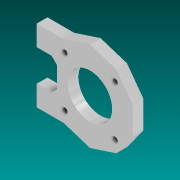
# Autodesk Inventor part: motorFrame
Saved by Autodesk Inventor 2020.2 (Build 242310000, 310)
## iProperties
Created: 2020-05-19
Part Number: motorFrame
Material: Aluminum 6061
Document SubType Name: Modeling
Designer: Svend
Density: 2.7 g/cm^3
Appearance: Aluminum - Polished
Author: Svend
Autodesk Inventor part; units mm, degrees
ref_plane "YZ Plane" through (0, 0, 0) normal (1, 0, 0) x (0, 1, 0)
ref_plane "XZ Plane" through (0, 0, 0) normal (0, 1, 0) x (-1, 0, 0)
ref_plane "XY Plane" through (0, 0, 0) normal (0, 0, 1) x (1, 0, 0)
ref_plane "Work Plane1" through (0, 0, 0) normal (0, 0, 1) x (1, 0, 0)
sketch "Sketch1" plane through (0, 0, 0) normal (0, 0, 1) x (1, 0, 0)
  circle A0 centre (0, 0) radius 21 projected
  circle A1 centre (23.57, -23.57) radius 2 projected
  circle A2 centre (23.57, 23.57) radius 2 projected
  circle A3 centre (-23.57, -23.57) radius 2.5 projected
  circle A4 centre (-23.57, 23.57) radius 2 projected
  circle A5 centre (-23.57, -23.57) radius 2 projected
  circle A6 centre (0, 0) radius 19 projected
  circle A7 centre (-23.57, 23.57) radius 2.5 projected
  circle A8 centre (-23.57, -23.57) radius 2.5 projected
  arc A9 (-29.95, -24.95) -> (-24.95, -29.95) centre (-24.95, -24.95) ccw projected
  line L0 (24.95, -29.95) -> (-24.95, -29.95) projected
  arc A10 (24.95, -29.95) -> (29.95, -24.95) centre (24.95, -24.95) ccw projected
  line L1 (29.95, 24.95) -> (29.95, -24.95) projected
  arc A11 (29.95, 24.95) -> (24.95, 29.95) centre (24.95, 24.95) ccw projected
  line L2 (-24.95, 29.95) -> (24.95, 29.95) projected
  arc A12 (-24.95, 29.95) -> (-29.95, 24.95) centre (-24.95, 24.95) ccw projected
  line L3 (-29.95, -24.95) -> (-29.95, 24.95) projected
  circle A13 centre (23.57, -23.57) radius 2.5 projected
  circle A14 centre (23.57, 23.57) radius 2.5 projected
  line L4 (-49.95, -90) -> (-49.95, 90) projected
  line L5 (-59.95, -90) -> (-49.95, -90)
  line L6 (-59.95, 90) -> (-49.95, 90)
  line L7 (40.2846, 0) -> (-40.2846, 0)
  line L8 (-49.95, -90) -> (-49.95, 90) projected
  line L9 (-59.95, -90) -> (-49.95, -90)
  line L10 (-49.95, 35.5095) -> (-26.95, 35.5095) projected
  line L11 (-24.95, 29.95) -> (-49.95, 29.95)
  line L12 (-24.95, -29.95) -> (-49.95, -29.95)
  circle A15 centre (0, 0) radius 22
  line L13 (-32.95, 22) -> (-32.95, -22) projected
  line L14 (-30.95, -14.95) -> (-49.95, -14.95)
  line L15 (-30.95, 14.95) -> (-49.95, 14.95)
  line L16 (-30.95, -14.95) -> (-30.95, 14.95)
  line L17 (24.7214, -34.026) -> (0, -42.0585)
  line L18 (0, -42.0585) -> (-24.7214, -34.026)
  line L19 (-24.7214, -34.026) -> (-40, -12.9968)
  line L20 (-40, -12.9968) -> (-40, 12.9968)
  line L21 (-40, 12.9968) -> (-24.7214, 34.026)
  line L22 (-24.7214, 34.026) -> (0, 42.0585)
  line L23 (0, 42.0585) -> (24.7214, 34.026)
  line L24 (24.7214, 34.026) -> (40, 12.9968)
  line L25 (40, 12.9968) -> (40, -12.9968)
  line L26 (40, -12.9968) -> (24.7214, -34.026)
  line L27 (-24.7214, -34.026) -> (-49.95, -34.026)
  line L28 (-24.7214, 34.026) -> (-49.95, 34.026)
  point P0 (0, 0)
  point P1 (-23.2856, -45.1645)
  point P2 (-49.95, -75.9684)
  point P3 (-23.2856, 45.1645)
  point P4 (-49.95, -14.95)
  dimension "d9" = 1
  dimension "d10" = 15
  dimension "d11" = 15
  dimension "d12" = 1
  dimension "d13" = 40
  constraints: 42 end point, 7 horizontal, 5 parallel, 2 perpendicular, 1 centre point, 1 coincident, 1 midpoint, 1 point on line, 1 symmetric about line, 1 vertical, 30 other
  measures "d9" radial gap between concentric circles of A0 A15
  measures "d10" distance between parallel lines of L12 L14
  measures "d11" distance between parallel lines of L11 L15
  measures "d12" distance between parallel lines of L3 L16
  measures "d13" distance from line of L25 point (0, 0)
extrude "Extrusion1" add sketch "Sketch1" along normal blind 10 contours L7 A15 A0 | A0 L7 A15 | A15 L7 L3 A12 L2 A11 L1 | L7 L1 A10 L0 A9 L3 A15 | L7 L25 L26 L17 L18 L19 L12 L0 A10 L1 | L1 A11 L2 L11 L21 L22 L23 L24 L25 L7 | L7 L16 L15 L21 L11 A12 L3 | L3 A9 L12 L19 L14 L16 L7 | L19 L27 L4 L12 | L12 L4 L14 L19 | L21 L15 L4 L11 | L11 L4 L28 L21
chamfer "Chamfer1" distance 5 angle 45 2 edges at (-30.95, 14.95, 5) (-30.95, -14.95, 5)
sketch "Sketch2" plane through (-49.95, -34.026, 0) normal (-1, 0, 0) x (0, 0, 1)
  line L0 (0, 19.076) -> (0, 0) projected
  line L1 (0, 0) -> (10, 0) projected
  line L2 (10, 19.076) -> (10, 0) projected
  line L3 (0, 19.076) -> (10, 19.076) projected
  line L4 (0, 68.0521) -> (0, 48.976) projected
  line L5 (0, 48.976) -> (10, 48.976) projected
  line L6 (10, 68.0521) -> (10, 48.976) projected
  line L7 (0, 68.0521) -> (10, 68.0521) projected
  point P0 (0, 34.026)
  point P1 (5, 9.538)
  point P2 (5, 58.514)
  point P3 (5, 68.0521)
  point P4 (5, 19.076)
  point P5 (0, 9.538)
  point P6 (0, 58.514)
  constraints: 4 midpoint, 2 horizontal alignment, 2 vertical alignment
hole "Hole1" at (-49.95, 24.488, 5) at (-49.95, -24.488, 5) direction (1, 0, 0) diameter 4.917 depth 17.1 tip angle 118 thread size "M6x1" class "6H" standard "ISO Metric profile"
equation "\"d11\" = d10"
body "Solid1"
